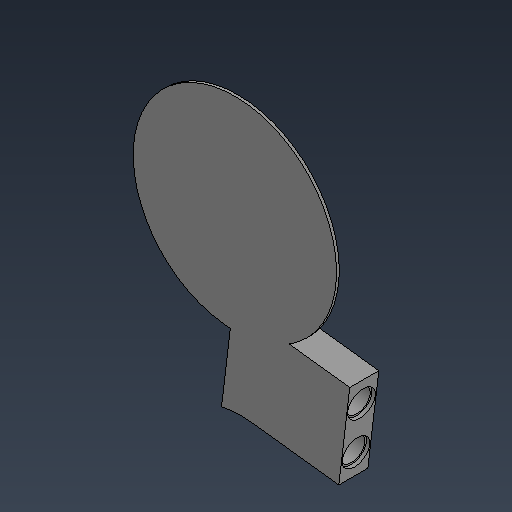
# Autodesk Inventor part: BearigHold
Saved by Autodesk Inventor 2026.2 (Build 302298010, 298A)
## iProperties
Created: 2026-04-04
Part Number: BearigHold
Material: Generic
Document SubType Name: Modeling
Designer: szymo
Density: 1 g/cm^3
Appearance: Default(1)
Author: szymo
Autodesk Inventor part; units mm, degrees
ref_plane "YZ Plane" through (0, 0, 0) normal (1, 0, 0) x (0, 1, 0)
ref_plane "XZ Plane" through (0, 0, 0) normal (0, 1, 0) x (-1, 0, 0)
ref_plane "XY Plane" through (0, 0, 0) normal (0, 0, 1) x (1, 0, 0)
ref_plane "Work Plane1" through (-1107.0645, 3929.3467, 0) normal (0, 0, 1) x (-0.9926876, 0.1207117, 0)
sketch "Sketch1" plane through (-1107.0645, 3929.3467, 0) normal (0, 0, 1) x (-0.9926876, 0.1207117, 0)
  circle A0 centre (14.5, -14.5) radius 13.85 projected
  circle A1 centre (14.5, -14.5) radius 14.5 projected
  circle A2 centre (14.5, -55.2958) radius 13.85 projected
  circle A3 centre (14.5, -55.2958) radius 14.5 projected
  circle A4 centre (13, -35.0012) radius 5 projected
  line L0 (0, 0) -> (29, 0)
  line L1 (29, 0) -> (29, -67)
  line L2 (29, -67) -> (0, -67)
  line L3 (0, -67) -> (0, 0)
  line L4 (2, 0) -> (2, -67)
  line L5 (14.5, -28.35) -> (2, -28.35)
  line L6 (14.5, -29) -> (2, -29)
  line L7 (14.5, -40.7958) -> (2, -40.7958)
  line L8 (14.5, -41.4458) -> (2, -41.4458)
  line L9 (19, 0) -> (19, -67)
  point P0 (-1573.2874, 3766.9781)
  point P1 (19, -42.1973)
  point P2 (19, -27.5986)
  point P3 (19, -41.5118)
  point P4 (19, -28.284)
  dimension "d0" = 67
  dimension "d1" = 2
  dimension "d2" = 1
  constraints: 20 end point, 8 point on line, 7 perpendicular, 5 horizontal, 2 parallel, 1 coincident, 1 vertical, 9 other
  measures "d0" distance of L2.end L0.start
  measures "d1" distance between parallel lines of L4 L3
  measures "d2" distance edge to line of A4 L9
ref_plane "Work Plane7" through (-17.5791, -32.927, 3.4) normal (0, 0, -1) x (0.0194385, 0.9998111, 0)
extrude "Extrusion1" add sketch "Sketch1" along normal blind 3.8 contours L9 A1 L5 A0 | L9 A3 L7 L4 L6 A1 | A1 L6 L4 L5 | L9 A2 L8 A3 | A3 L8 L4 L7
ref_plane "Work Plane8" through (-22.6017, 2.8462, 4) normal (0, 0, -1) x (0.4990785, 0.8665568, 0)
ref_plane "Work Plane9" through (151.4324, -161.9595, 4) normal (0, 0, 1) x (0.0950598, 0.9954716, 0)
sketch "Sketch2" plane through (-1107.0645, 3929.3467, 3.8) normal (0, 0, 1) x (0.9926876, -0.1207117, 0)
  arc A0 (-19, 42.1973) -> (-14.5, 41.4458) centre (-14.5, 55.2958) ccw projected
  line L0 (-19, 42.1973) -> (-19, 27.5986) projected
  arc A1 (-14.5, 28.35) -> (-19, 27.5986) centre (-14.5, 14.5) ccw projected
  line L1 (-14.5, 28.35) -> (-2, 28.35) projected
  line L2 (-2, 28.35) -> (-2, 41.4458) projected
  line L3 (-2, 41.4458) -> (-14.5, 41.4458) projected
  circle A2 centre (-13, 35.0012) radius 5 projected
  circle A3 centre (-20.1246, 52.8194) radius 14.7 projected
  line L4 (-20.1246, 38.1194) -> (-2, 38.1194)
  line L5 (-2, 28.35) -> (-2, 41.4458) projected
  line L6 (-20.1246, 52.8194) -> (-20.1246, 38.1194)
  point P0 (-2, 38.1194)
  point P1 (-19, 38.1625)
  point P2 (-10.8116, 41.4458)
  point P3 (-19, 38.1194)
  constraints: 4 end point, 2 perpendicular, 1 point on line, 2 other
extrude "Extrusion4" add sketch "Sketch2" along normal blind 0.4
sketch "Sketch3" plane through (-1105.6277, 3957.7308, 0) normal (0.9926876, -0.1207117, 0) x (0, 0, -1)
  line L0 (0, 0) -> (-4.2, 0) projected
  line L1 (0, 0) -> (0, 13.0958) projected
  line L2 (0, 13.0958) -> (-4.2, 13.0958) projected
  line L3 (-4.2, 6.5479) -> (0, 6.5479)
  line L4 (-4.2, 6.5479) -> (0, 0)
  line L5 (-4.2, 6.5479) -> (0, 13.0958)
  line L6 (0, 6.5479) -> (-2.1, 9.8219)
  line L7 (0, 6.5479) -> (-2.1, 3.274)
  line L8 (-4.2, 0) -> (-4.2, 13.0958) projected
  point P0 (0, -3795.3281)
  dimension "d11" = 6.5479
  dimension "d12" = 6.5479
  constraints: 10 end point, 4 midpoint, 2 coincident, 1 perpendicular
  measures "d11" distance between parallel lines of L0 L3
  measures "d12" distance between parallel lines of L2 L3
hole "Hole1" at (-1105.2325, 3960.9809, 2.1) at (-1104.4421, 3967.4809, 2.1) direction (-0.9926876, 0.1207117, 0) diameter 3.5 depth 4.5 counterbore diameter 4 counterbore depth 0.5
equation "\"d11\" = d12"
body "Solid1"
